Autodesk Inventor part; units mm, degrees
(part 3 of 3)
sketch "Sketch12" plane through (0, 0, 6.35) normal (0, 0, 1) x (1, 0, 0)
  line L0 (-36.4792, -134.4184) -> (-53.8135, -133.1797) projected
  line L1 (-53.8135, -133.1797) -> (-84.6539, -130.9759)
  arc A0 (-85.584, -139.4585) -> (-93.4457, -121.7087) centre (-97.0281, -133.9113) ccw projected
  arc A1 (-79.0435, -94.0873) -> (-76.0538, -98.0209) centre (-69.1823, -89.6953) ccw projected
  line L2 (-76.0538, -98.0209) -> (-35.3556, -131.6106) projected
  arc A2 (-36.4792, -134.4184) -> (-35.3556, -131.6106) centre (-36.3661, -132.835) ccw projected
  line L3 (-36.4792, -134.4184) -> (-53.8135, -133.1797) projected
  arc A3 (-53.8135, -133.1797) -> (-74.1957, -134.2859) centre (-63.595, -141.2799) ccw projected
  spline S0 degree 4 poles (-74.1957, -134.2859) (-76.3935, -137.6171) (-78.0776, -144.0197) (-82.6045, -141.2731) (-85.584, -139.4585) knots 0 0 0 0 0 1 1 1 1 1 projected
  arc A4 (-85.584, -139.4585) -> (-93.4457, -121.7087) centre (-97.0281, -133.9113) ccw projected
  line L4 (-93.4457, -121.7087) -> (-88.3648, -96.7304) projected
  arc A5 (-88.3648, -96.7304) -> (-79.0435, -94.0873) centre (-86.902, -84.1308) ccw projected
  arc A6 (-57.0315, -170.4891) -> (-48.9168, -167.9529) centre (-56.5442, -157.7985) ccw projected
  arc A7 (-45.5693, -167.6622) -> (-48.9168, -167.9529) centre (-47.0099, -170.4916) ccw projected
  line L5 (-45.5693, -167.6622) -> (-40.3949, -170.2969) projected
  arc A8 (-39.0062, -174.5669) -> (-40.3949, -170.2969) centre (-41.8356, -173.1263) ccw projected
  line L6 (-39.0062, -174.5669) -> (-46.1931, -188.6814) projected
  arc A9 (-49.6531, -190.3525) -> (-46.1931, -188.6814) centre (-49.0224, -187.2408) ccw projected
  arc A10 (-49.6531, -190.3525) -> (-53.7154, -190.1932) centre (-52.1756, -202.7997) ccw projected
  arc A11 (-56.7611, -188.774) -> (-53.7154, -190.1932) centre (-54.1004, -187.0416) ccw projected
  line L7 (-56.7611, -188.774) -> (-63.6057, -178.2615) projected
  line L8 (-44.8637, -152.8128) -> (-47.8206, -145.8856) projected
  arc A12 (-44.6741, -141.4723) -> (-47.8206, -145.8856) centre (-44.9004, -144.6392) ccw projected
  line L9 (-44.6741, -141.4723) -> (-34.3957, -142.2068) projected
  arc A13 (-31.6785, -144.1834) -> (-34.3957, -142.2068) centre (-34.622, -145.3737) ccw projected
  arc A14 (-31.6785, -144.1834) -> (-28.4869, -148.7838) centre (-19.9049, -139.4226) ccw projected
  arc A15 (-27.8031, -152.5648) -> (-28.4869, -148.7838) centre (-30.6324, -151.1242) ccw projected
  line L10 (-27.8031, -152.5648) -> (-32.6673, -162.1179) projected
  arc A16 (-36.9373, -163.5065) -> (-32.6673, -162.1179) centre (-35.4967, -160.6772) ccw projected
  line L11 (-36.9373, -163.5065) -> (-42.1117, -160.8718) projected
  arc A17 (-43.8457, -157.9937) -> (-42.1117, -160.8718) centre (-40.6711, -158.0425) ccw projected
  arc A18 (-43.8457, -157.9937) -> (-44.8637, -152.8128) centre (-56.5442, -157.7985) ccw projected
  arc A19 (-88.6501, -203.823) -> (-105.4512, -206.2136) centre (-93.207, -232.0324) ccw projected
  arc A20 (-109.9229, -202.7119) -> (-105.4512, -206.2136) centre (-106.8116, -203.3448) ccw projected
  line L12 (-109.9229, -202.7119) -> (-109.1463, -198.894) projected
  arc A21 (-106.2582, -196.3597) -> (-109.1463, -198.894) centre (-106.035, -199.5269) ccw projected
  arc A22 (-106.2582, -196.3597) -> (-98.2131, -192.7137) centre (-107.1508, -183.6911) ccw projected
  arc A23 (-94.9362, -191.9703) -> (-98.2131, -192.7137) centre (-95.9786, -194.9693) ccw projected
  line L13 (-94.9362, -191.9703) -> (-86.0453, -195.0607) projected
  arc A24 (-84.1415, -199.2432) -> (-86.0453, -195.0607) centre (-87.0877, -198.0597) ccw projected
  line L14 (-84.1415, -199.2432) -> (-85.1976, -201.8722) projected
  arc A25 (-88.6501, -203.823) -> (-85.1976, -201.8722) centre (-88.1438, -200.6887) ccw projected
  arc A26 (-28.8338, -52.5675) -> (-24.5423, -50.875) centre (-27.4885, -49.6916) ccw projected
  line L15 (-28.8338, -52.5675) -> (-62.2455, -36.9386) projected
  arc A27 (-64.0747, -34.1201) -> (-62.2455, -36.9386) centre (-60.9002, -34.0627) ccw projected
  arc A28 (-64.0747, -34.1201) -> (-69.5394, -23.9106) centre (-76.7726, -34.3495) ccw projected
  arc A29 (-70.5555, -19.8506) -> (-69.5394, -23.9106) centre (-67.7311, -21.3009) ccw projected
  arc A30 (-64.7921, -10.8233) -> (-70.5555, -19.8506) centre (-19.7161, -45.9556) ccw projected
  line L16 (-64.7921, -10.8233) -> (-52.5862, 4.8373) projected
  arc A31 (-46.9122, 2.7029) -> (-52.5862, 4.8373) centre (-50.0819, 2.8855) ccw projected
  arc A32 (-46.9122, 2.7029) -> (-23.4162, -40.7399) centre (0, 0) ccw projected
  arc A33 (-22.0522, -44.6761) -> (-23.4162, -40.7399) centre (-24.9984, -43.4926) ccw projected
  line L17 (-22.0522, -44.6761) -> (-24.5423, -50.875) projected
  arc A34 (-88.5384, -146.9458) -> (-92.3643, -145.7246) centre (-91.1992, -148.6781) ccw projected
  line L18 (-88.5384, -146.9458) -> (-60.6619, -189.7645) projected
  arc A35 (-61.0933, -193.7573) -> (-60.6619, -189.7645) centre (-63.3227, -191.4968) ccw projected
  arc A36 (-61.0933, -193.7573) -> (-61.1133, -193.7771) centre (-52.1756, -202.7997) ccw projected
  arc A37 (-64.3902, -194.5205) -> (-61.1133, -193.7771) centre (-63.3478, -191.5215) ccw projected
  line L19 (-64.3902, -194.5205) -> (-92.4345, -184.7727) projected
  arc A38 (-94.5438, -182.1572) -> (-92.4345, -184.7727) centre (-91.3921, -181.7737) ccw projected
  arc A39 (-94.5438, -182.1572) -> (-101.38, -172.378) centre (-107.1508, -183.6911) ccw projected
  arc A40 (-103.0485, -168.9169) -> (-101.38, -172.378) centre (-99.9372, -169.5497) ccw projected
  line L20 (-103.0485, -168.9169) -> (-99.0202, -149.1135) projected
  arc A41 (-96.1321, -146.5792) -> (-99.0202, -149.1135) centre (-95.909, -149.7463) ccw projected
  arc A42 (-96.1321, -146.5792) -> (-92.3643, -145.7246) centre (-97.0248, -133.9106) ccw projected
  arc A43 (-17.7611, -54.4364) -> (-16.1602, -58.4958) centre (-14.8149, -55.6198) ccw projected
  line L21 (-17.7611, -54.4364) -> (-14.9814, -47.5164) projected
  arc A44 (-11.2735, -45.6176) -> (-14.9814, -47.5164) centre (-12.0352, -48.6999) ccw projected
  arc A45 (-11.2735, -45.6176) -> (22.3352, -41.3425) centre (0, 0) ccw projected
  arc A46 (26.6737, -45.5765) -> (22.3352, -41.3425) centre (23.8443, -44.1359) ccw projected
  line L22 (26.6737, -45.5765) -> (18.3481, -61.9274) projected
  arc A47 (14.8881, -63.5984) -> (18.3481, -61.9274) centre (15.5187, -60.4867) ccw projected
  arc A48 (14.8881, -63.5984) -> (4.4031, -66.1517) centre (12.3657, -76.0454) ccw projected
  arc A49 (1.0672, -66.5541) -> (4.4031, -66.1517) centre (2.4124, -63.6782) ccw projected
  line L23 (1.0672, -66.5541) -> (-16.1602, -58.4958) projected
  arc A50 (-75.9854, -77.6347) -> (-81.1278, -72.8169) centre (-86.8987, -84.1301) ccw projected
  arc A51 (-82.7964, -69.3558) -> (-81.1278, -72.8169) centre (-79.6851, -69.9886) ccw projected
  line L24 (-82.7964, -69.3558) -> (-78.7681, -49.5524) projected
  arc A52 (-75.88, -47.0181) -> (-78.7681, -49.5524) centre (-75.6568, -50.1853) ccw projected
  arc A53 (-75.88, -47.0181) -> (-68.81, -44.2433) centre (-76.7726, -34.3495) ccw projected
  arc A54 (-65.4741, -43.8408) -> (-68.81, -44.2433) centre (-66.8194, -46.7167) ccw projected
  line L25 (-65.4741, -43.8408) -> (-13.0902, -68.3442) projected
  arc A55 (-14.1778, -74.3847) -> (-13.0902, -68.3442) centre (-14.4355, -71.2201) ccw projected
  line L26 (-14.1778, -74.3847) -> (-72.9993, -79.1754) projected
  arc A56 (-75.9854, -77.6347) -> (-72.9993, -79.1754) centre (-73.2571, -76.0109) ccw projected
  arc A57 (1.4524, -82.5408) -> (3.7836, -85.4069) centre (12.3657, -76.0454) ccw projected
  arc A58 (4.4674, -89.1879) -> (3.7836, -85.4069) centre (1.6381, -87.7473) ccw projected
  line L27 (4.4674, -89.1879) -> (-13.9226, -125.3045) projected
  arc A59 (-17.3825, -126.9756) -> (-13.9226, -125.3045) centre (-16.7519, -123.8638) ccw projected
  arc A60 (-17.3825, -126.9756) -> (-25.1437, -127.8534) centre (-19.9049, -139.4226) ccw projected
  arc A61 (-28.4744, -127.4098) -> (-25.1437, -127.8534) centre (-26.4534, -124.9611) ccw projected
  line L28 (-28.4744, -127.4098) -> (-71.2033, -92.144) projected
  arc A62 (-69.4401, -86.5307) -> (-71.2033, -92.144) centre (-69.1823, -89.6953) ccw projected
  line L29 (-69.4401, -86.5307) -> (-1.5337, -81.0001) projected
  arc A63 (1.4524, -82.5408) -> (-1.5337, -81.0001) centre (-1.2759, -84.1646) ccw projected
  arc A64 (-64.7826, -204.3336) -> (-60.7577, -212.1612) centre (-52.1756, -202.7997) ccw projected
  arc A65 (-60.0739, -215.9422) -> (-60.7577, -212.1612) centre (-62.9032, -214.5015) ccw projected
  line L30 (-60.0739, -215.9422) -> (-61.8764, -219.4822) projected
  arc A66 (-67.5559, -219.4407) -> (-61.8764, -219.4822) centre (-64.7057, -218.0416) ccw projected
  arc A67 (-67.5559, -219.4407) -> (-76.9832, -208.5096) centre (-93.207, -232.0324) ccw projected
  arc A68 (-78.1267, -204.7125) -> (-76.9832, -208.5096) centre (-75.1805, -205.896) ccw projected
  line L31 (-78.1267, -204.7125) -> (-76.8234, -201.468) projected
  arc A69 (-72.8348, -199.6524) -> (-76.8234, -201.468) centre (-73.8772, -202.6514) ccw projected
  line L32 (-72.8348, -199.6524) -> (-66.8919, -201.7181) projected
  arc A70 (-64.7826, -204.3336) -> (-66.8919, -201.7181) centre (-67.9343, -204.7171) ccw projected
  circle A71 centre (-19.9049, -139.4226) radius 5.588 projected
  circle A72 centre (-107.1541, -183.6919) radius 5.588 projected
  circle A73 centre (-86.902, -84.1308) radius 5.588 projected
  circle A74 centre (-56.5442, -157.7985) radius 6.731 projected
  line L33 (-98.5201, -236.7413) -> (-93.7862, -224.9565) projected
  arc A75 (-87.8938, -227.3235) -> (-93.7862, -224.9565) centre (-90.84, -226.14) ccw projected
  line L34 (-87.8938, -227.3235) -> (-92.6277, -239.1082) projected
  arc A76 (-98.5201, -236.7413) -> (-92.6277, -239.1082) centre (-95.5739, -237.9247) ccw projected
  circle A77 centre (0, 0) radius 13.4937 projected
  arc A78 (56.5867, -28.8131) -> (-50.0844, 39.0359) centre (0, 0) ccw projected
  line L35 (-50.0844, 39.0359) -> (-79.8174, 0.8875) projected
  arc A79 (-79.8174, 0.8875) -> (-94.3869, -30.7665) centre (-19.7161, -45.9556) ccw projected
  line L36 (-94.3869, -30.7665) -> (-133.6537, -223.8049) projected
  arc A80 (-133.6537, -223.8049) -> (-56.4256, -250.7609) centre (-93.207, -232.0324) ccw projected
  line L37 (-56.4256, -250.7609) -> (56.5867, -28.8131) projected
  circle A81 centre (-63.595, -141.2799) radius 6.731 projected
  arc A82 (-11.6087, -28.8683) -> (-9.2396, -22.9769) centre (-10.4059, -25.9299) ccw projected
  arc A83 (-9.2396, -22.9769) -> (-11.6087, -28.8683) centre (-10.4424, -25.9152) ccw projected
  arc A84 (26.36, 16.5315) -> (20.9805, 13.1578) centre (23.6598, 14.8613) ccw projected
  arc A85 (20.9805, 13.1578) -> (26.36, 16.5315) centre (23.6807, 14.828) ccw projected
  arc A86 (23.8681, -19.9613) -> (18.9971, -15.8876) centre (21.4452, -17.9094) ccw projected
  arc A87 (18.9971, -15.8876) -> (23.8681, -19.9613) centre (21.42, -17.9396) ccw projected
  arc A88 (-7.5767, 30.1783) -> (-6.0305, 24.0196) centre (-6.8227, 27.0942) ccw projected
  arc A89 (-6.0305, 24.0196) -> (-7.5767, 30.1783) centre (-6.7845, 27.1038) ccw projected
  arc A90 (-31.0426, 2.1197) -> (-24.7075, 1.6871) centre (-27.8764, 1.8838) ccw projected
  arc A91 (-24.7075, 1.6871) -> (-31.0426, 2.1197) centre (-27.8737, 1.9231) ccw projected
  circle A92 centre (-76.7759, -34.3502) radius 5.588 projected
  circle A93 centre (-97.0281, -133.9113) radius 5.588 projected
  circle A94 centre (12.3657, -76.0454) radius 5.588 projected
  circle A95 centre (-52.1756, -202.7997) radius 5.588 projected
  point P0 (0, 0)
  point P1 (-85.584, -139.4585)
  point P2 (-72.1254, -131.8712)
  constraints: 2 end point, 1 collinear, 1 point on circle, 2 other
extrude "Extrusion12" add sketch "Sketch12" against normal blind 6.35 contours A3 S0 A0 L1
fillet "Fillet2" radius 3.175 6 edges at (-93.4457, -121.7087, 3.175) (-84.6539, -130.9759, 3.175) (-79.0435, -94.0873, 3.175) (-88.3648, -96.7304, 3.175) (-72.1254, -131.8712, 3.175) (-53.8135, -133.1797, 3.175)
sketch "Sketch13" plane through (0, 0, 6.35) normal (0, 0, 1) x (1, 0, 0)
  circle A0 centre (-97.0281, -133.9113) radius 2.413 projected
  circle A1 centre (-52.1756, -202.7997) radius 2.413 projected
  line L0 (-97.0281, -133.9113) -> (-52.1756, -202.7997)
  line L1 (-100.2209, -135.9902) -> (-55.3728, -204.8718)
  arc A2 (-77.598, -96.456) -> (-76.0538, -98.0209) centre (-69.1823, -89.6953) ccw projected
  line L2 (-76.0538, -98.0209) -> (-35.3556, -131.6106) projected
  arc A3 (-36.4792, -134.4184) -> (-35.3556, -131.6106) centre (-36.3661, -132.835) ccw projected
  line L3 (-36.4792, -134.4184) -> (-52.5475, -133.2702) projected
  arc A4 (-54.5759, -132.3386) -> (-52.5475, -133.2702) centre (-52.3212, -130.1033) ccw projected
  arc A5 (-54.5759, -132.3386) -> (-71.2511, -131.147) centre (-63.595, -141.2799) ccw projected
  arc A6 (-73.3914, -131.7807) -> (-71.2511, -131.147) centre (-73.1651, -128.6138) ccw projected
  line L4 (-73.3914, -131.7807) -> (-82.5175, -131.1285) projected
  arc A7 (-85.2353, -129.1502) -> (-82.5175, -131.1285) centre (-82.2912, -127.9616) ccw projected
  arc A8 (-85.2353, -129.1502) -> (-91.2504, -122.5819) centre (-97.0281, -133.9113) ccw projected
  arc A9 (-92.9193, -119.1206) -> (-91.2504, -122.5819) centre (-89.808, -119.7535) ccw projected
  line L5 (-92.9193, -119.1206) -> (-88.891, -99.3174) projected
  arc A10 (-86.0044, -96.7832) -> (-88.891, -99.3174) centre (-85.7797, -99.9502) ccw projected
  arc A11 (-86.0044, -96.7832) -> (-81.4403, -95.5789) centre (-86.902, -84.1308) ccw projected
  arc A12 (-77.598, -96.456) -> (-81.4403, -95.5789) centre (-80.0732, -98.4445) ccw projected
  arc A13 (-57.0315, -170.4891) -> (-48.9168, -167.9529) centre (-56.5442, -157.7985) ccw projected
  arc A14 (-45.5693, -167.6622) -> (-48.9168, -167.9529) centre (-47.0099, -170.4916) ccw projected
  line L6 (-45.5693, -167.6622) -> (-40.3949, -170.2969) projected
  arc A15 (-39.0062, -174.5669) -> (-40.3949, -170.2969) centre (-41.8356, -173.1263) ccw projected
  line L7 (-39.0062, -174.5669) -> (-46.1931, -188.6814) projected
  arc A16 (-49.6531, -190.3525) -> (-46.1931, -188.6814) centre (-49.0224, -187.2408) ccw projected
  arc A17 (-49.6531, -190.3525) -> (-53.7154, -190.1932) centre (-52.1756, -202.7997) ccw projected
  arc A18 (-56.7611, -188.774) -> (-53.7154, -190.1932) centre (-54.1004, -187.0416) ccw projected
  line L8 (-56.7611, -188.774) -> (-63.6057, -178.2615) projected
  line L9 (-44.8637, -152.8128) -> (-47.8206, -145.8856) projected
  arc A19 (-44.6741, -141.4723) -> (-47.8206, -145.8856) centre (-44.9004, -144.6392) ccw projected
  line L10 (-44.6741, -141.4723) -> (-34.3957, -142.2068) projected
  arc A20 (-31.6785, -144.1834) -> (-34.3957, -142.2068) centre (-34.622, -145.3737) ccw projected
  arc A21 (-31.6785, -144.1834) -> (-28.4869, -148.7838) centre (-19.9049, -139.4226) ccw projected
  arc A22 (-27.8031, -152.5648) -> (-28.4869, -148.7838) centre (-30.6324, -151.1242) ccw projected
  line L11 (-27.8031, -152.5648) -> (-32.6673, -162.1179) projected
  arc A23 (-36.9373, -163.5065) -> (-32.6673, -162.1179) centre (-35.4967, -160.6772) ccw projected
  line L12 (-36.9373, -163.5065) -> (-42.1117, -160.8718) projected
  arc A24 (-43.8457, -157.9937) -> (-42.1117, -160.8718) centre (-40.6711, -158.0425) ccw projected
  arc A25 (-43.8457, -157.9937) -> (-44.8637, -152.8128) centre (-56.5442, -157.7985) ccw projected
  arc A26 (-88.6501, -203.823) -> (-105.4512, -206.2136) centre (-93.207, -232.0324) ccw projected
  arc A27 (-109.9229, -202.7119) -> (-105.4512, -206.2136) centre (-106.8116, -203.3448) ccw projected
  line L13 (-109.9229, -202.7119) -> (-109.1463, -198.894) projected
  arc A28 (-106.2582, -196.3597) -> (-109.1463, -198.894) centre (-106.035, -199.5269) ccw projected
  arc A29 (-106.2582, -196.3597) -> (-98.2131, -192.7137) centre (-107.1508, -183.6911) ccw projected
  arc A30 (-94.9362, -191.9703) -> (-98.2131, -192.7137) centre (-95.9786, -194.9693) ccw projected
  line L14 (-94.9362, -191.9703) -> (-86.0453, -195.0607) projected
  arc A31 (-84.1415, -199.2432) -> (-86.0453, -195.0607) centre (-87.0877, -198.0597) ccw projected
  line L15 (-84.1415, -199.2432) -> (-85.1976, -201.8722) projected
  arc A32 (-88.6501, -203.823) -> (-85.1976, -201.8722) centre (-88.1438, -200.6887) ccw projected
  arc A33 (-28.8338, -52.5675) -> (-24.5423, -50.875) centre (-27.4885, -49.6916) ccw projected
  line L16 (-28.8338, -52.5675) -> (-62.2455, -36.9386) projected
  arc A34 (-64.0747, -34.1201) -> (-62.2455, -36.9386) centre (-60.9002, -34.0627) ccw projected
  arc A35 (-64.0747, -34.1201) -> (-69.5394, -23.9106) centre (-76.7726, -34.3495) ccw projected
  arc A36 (-70.5555, -19.8506) -> (-69.5394, -23.9106) centre (-67.7311, -21.3009) ccw projected
  arc A37 (-64.7921, -10.8233) -> (-70.5555, -19.8506) centre (-19.7161, -45.9556) ccw projected
  line L17 (-64.7921, -10.8233) -> (-52.5862, 4.8373) projected
  arc A38 (-46.9122, 2.7029) -> (-52.5862, 4.8373) centre (-50.0819, 2.8855) ccw projected
  arc A39 (-46.9122, 2.7029) -> (-23.4162, -40.7399) centre (0, 0) ccw projected
  arc A40 (-22.0522, -44.6761) -> (-23.4162, -40.7399) centre (-24.9984, -43.4926) ccw projected
  line L18 (-22.0522, -44.6761) -> (-24.5423, -50.875) projected
  arc A41 (-88.5384, -146.9458) -> (-92.3643, -145.7246) centre (-91.1992, -148.6781) ccw projected
  line L19 (-88.5384, -146.9458) -> (-60.6619, -189.7645) projected
  arc A42 (-61.0933, -193.7573) -> (-60.6619, -189.7645) centre (-63.3227, -191.4968) ccw projected
  arc A43 (-61.0933, -193.7573) -> (-61.1133, -193.7771) centre (-52.1756, -202.7997) ccw projected
  arc A44 (-64.3902, -194.5205) -> (-61.1133, -193.7771) centre (-63.3478, -191.5215) ccw projected
  line L20 (-64.3902, -194.5205) -> (-92.4345, -184.7727) projected
  arc A45 (-94.5438, -182.1572) -> (-92.4345, -184.7727) centre (-91.3921, -181.7737) ccw projected
  arc A46 (-94.5438, -182.1572) -> (-101.38, -172.378) centre (-107.1508, -183.6911) ccw projected
  arc A47 (-103.0485, -168.9169) -> (-101.38, -172.378) centre (-99.9372, -169.5497) ccw projected
  line L21 (-103.0485, -168.9169) -> (-99.0202, -149.1135) projected
  arc A48 (-96.1321, -146.5792) -> (-99.0202, -149.1135) centre (-95.909, -149.7463) ccw projected
  arc A49 (-96.1321, -146.5792) -> (-92.3643, -145.7246) centre (-97.0248, -133.9106) ccw projected
  arc A50 (-17.7611, -54.4364) -> (-16.1602, -58.4958) centre (-14.8149, -55.6198) ccw projected
  line L22 (-17.7611, -54.4364) -> (-14.9814, -47.5164) projected
  arc A51 (-11.2735, -45.6176) -> (-14.9814, -47.5164) centre (-12.0352, -48.6999) ccw projected
  arc A52 (-11.2735, -45.6176) -> (22.3352, -41.3425) centre (0, 0) ccw projected
  arc A53 (26.6737, -45.5765) -> (22.3352, -41.3425) centre (23.8443, -44.1359) ccw projected
  line L23 (26.6737, -45.5765) -> (18.3481, -61.9274) projected
  arc A54 (14.8881, -63.5984) -> (18.3481, -61.9274) centre (15.5187, -60.4867) ccw projected
  arc A55 (14.8881, -63.5984) -> (4.4031, -66.1517) centre (12.3657, -76.0454) ccw projected
  arc A56 (1.0672, -66.5541) -> (4.4031, -66.1517) centre (2.4124, -63.6782) ccw projected
  line L24 (1.0672, -66.5541) -> (-16.1602, -58.4958) projected
  arc A57 (-75.9854, -77.6347) -> (-81.1278, -72.8169) centre (-86.8987, -84.1301) ccw projected
  arc A58 (-82.7964, -69.3558) -> (-81.1278, -72.8169) centre (-79.6851, -69.9886) ccw projected
  line L25 (-82.7964, -69.3558) -> (-78.7681, -49.5524) projected
  arc A59 (-75.88, -47.0181) -> (-78.7681, -49.5524) centre (-75.6568, -50.1853) ccw projected
  arc A60 (-75.88, -47.0181) -> (-68.81, -44.2433) centre (-76.7726, -34.3495) ccw projected
  arc A61 (-65.4741, -43.8408) -> (-68.81, -44.2433) centre (-66.8194, -46.7167) ccw projected
  line L26 (-65.4741, -43.8408) -> (-13.0902, -68.3442) projected
  arc A62 (-14.1778, -74.3847) -> (-13.0902, -68.3442) centre (-14.4355, -71.2201) ccw projected
  line L27 (-14.1778, -74.3847) -> (-72.9993, -79.1754) projected
  arc A63 (-75.9854, -77.6347) -> (-72.9993, -79.1754) centre (-73.2571, -76.0109) ccw projected
  arc A64 (1.4524, -82.5408) -> (3.7836, -85.4069) centre (12.3657, -76.0454) ccw projected
  arc A65 (4.4674, -89.1879) -> (3.7836, -85.4069) centre (1.6381, -87.7473) ccw projected
  line L28 (4.4674, -89.1879) -> (-13.9226, -125.3045) projected
  arc A66 (-17.3825, -126.9756) -> (-13.9226, -125.3045) centre (-16.7519, -123.8638) ccw projected
  arc A67 (-17.3825, -126.9756) -> (-25.1437, -127.8534) centre (-19.9049, -139.4226) ccw projected
  arc A68 (-28.4744, -127.4098) -> (-25.1437, -127.8534) centre (-26.4534, -124.9611) ccw projected
  line L29 (-28.4744, -127.4098) -> (-71.2033, -92.144) projected
  arc A69 (-69.4401, -86.5307) -> (-71.2033, -92.144) centre (-69.1823, -89.6953) ccw projected
  line L30 (-69.4401, -86.5307) -> (-1.5337, -81.0001) projected
  arc A70 (1.4524, -82.5408) -> (-1.5337, -81.0001) centre (-1.2759, -84.1646) ccw projected
  arc A71 (-64.7826, -204.3336) -> (-60.7577, -212.1612) centre (-52.1756, -202.7997) ccw projected
  arc A72 (-60.0739, -215.9422) -> (-60.7577, -212.1612) centre (-62.9032, -214.5015) ccw projected
  line L31 (-60.0739, -215.9422) -> (-61.8764, -219.4822) projected
  arc A73 (-67.5559, -219.4407) -> (-61.8764, -219.4822) centre (-64.7057, -218.0416) ccw projected
  arc A74 (-67.5559, -219.4407) -> (-76.9832, -208.5096) centre (-93.207, -232.0324) ccw projected
  arc A75 (-78.1267, -204.7125) -> (-76.9832, -208.5096) centre (-75.1805, -205.896) ccw projected
  line L32 (-78.1267, -204.7125) -> (-76.8234, -201.468) projected
  arc A76 (-72.8348, -199.6524) -> (-76.8234, -201.468) centre (-73.8772, -202.6514) ccw projected
  line L33 (-72.8348, -199.6524) -> (-66.8919, -201.7181) projected
  arc A77 (-64.7826, -204.3336) -> (-66.8919, -201.7181) centre (-67.9343, -204.7171) ccw projected
  circle A78 centre (-19.9049, -139.4226) radius 5.588 projected
  circle A79 centre (-107.1541, -183.6919) radius 5.588 projected
  circle A80 centre (-86.902, -84.1308) radius 5.588 projected
  circle A81 centre (-56.5442, -157.7985) radius 6.731 projected
  line L34 (-98.5201, -236.7413) -> (-93.7862, -224.9565) projected
  arc A82 (-87.8938, -227.3235) -> (-93.7862, -224.9565) centre (-90.84, -226.14) ccw projected
  line L35 (-87.8938, -227.3235) -> (-92.6277, -239.1082) projected
  arc A83 (-98.5201, -236.7413) -> (-92.6277, -239.1082) centre (-95.5739, -237.9247) ccw projected
  circle A84 centre (0, 0) radius 13.4937 projected
  arc A85 (56.5867, -28.8131) -> (-50.0844, 39.0359) centre (0, 0) ccw projected
  line L36 (-50.0844, 39.0359) -> (-79.8174, 0.8875) projected
  arc A86 (-79.8174, 0.8875) -> (-94.3869, -30.7665) centre (-19.7161, -45.9556) ccw projected
  line L37 (-94.3869, -30.7665) -> (-133.6537, -223.8049) projected
  arc A87 (-133.6537, -223.8049) -> (-56.4256, -250.7609) centre (-93.207, -232.0324) ccw projected
  line L38 (-56.4256, -250.7609) -> (56.5867, -28.8131) projected
  circle A88 centre (-63.595, -141.2799) radius 6.731 projected
  arc A89 (-11.6087, -28.8683) -> (-9.2396, -22.9769) centre (-10.4059, -25.9299) ccw projected
  arc A90 (-9.2396, -22.9769) -> (-11.6087, -28.8683) centre (-10.4424, -25.9152) ccw projected
  arc A91 (26.36, 16.5315) -> (20.9805, 13.1578) centre (23.6598, 14.8613) ccw projected
  arc A92 (20.9805, 13.1578) -> (26.36, 16.5315) centre (23.6807, 14.828) ccw projected
  arc A93 (23.8681, -19.9613) -> (18.9971, -15.8876) centre (21.4452, -17.9094) ccw projected
  arc A94 (18.9971, -15.8876) -> (23.8681, -19.9613) centre (21.42, -17.9396) ccw projected
  arc A95 (-7.5767, 30.1783) -> (-6.0305, 24.0196) centre (-6.8227, 27.0942) ccw projected
  arc A96 (-6.0305, 24.0196) -> (-7.5767, 30.1783) centre (-6.7845, 27.1038) ccw projected
  arc A97 (-31.0426, 2.1197) -> (-24.7075, 1.6871) centre (-27.8764, 1.8838) ccw projected
  arc A98 (-24.7075, 1.6871) -> (-31.0426, 2.1197) centre (-27.8737, 1.9231) ccw projected
  circle A99 centre (-76.7759, -34.3502) radius 5.588 projected
  circle A100 centre (-97.0281, -133.9113) radius 5.588 projected
  circle A101 centre (12.3657, -76.0454) radius 5.588 projected
  circle A102 centre (-52.1756, -202.7997) radius 5.588 projected
  point P0 (0, 0)
  point P1 (-93.6105, -146.1431)
  point P2 (-62.1505, -194.4621)
  dimension "d55" = 3.81
  constraints: 4 end point, 1 parallel, 1 other
  measures "d55" distance between parallel lines of L0 L1
extrude "Extrusion13" add sketch "Sketch13" against normal blind 6.35 contours A41 L19 L0 | L0 A42 A43 A44 L1 A49 A41
fillet "Fillet3" radius 3.175 2 edges at (-93.6105, -146.1431, 3.175) (-62.1505, -194.4621, 3.175)
body "Solid1"
